Slidercrank (Autodesk Fusion 360 design; units mm, degrees)
Autodesk Fusion 360 part; units mm, degrees
note: some values were not read from the file. Set by a fixed rule: which sketch regions a step uses.
sketch "Sketch2" plane through (0, 0, 0) normal (0, 1, 0) x (1, 0, 0) in component "Bottom"
  circle A0 centre (0, 0) radius 42.5
  dimension "d1" = 85
  constraint coincident A0.centre origin
  measures "d1" diameter of A0
extrude "Extrude1" add sketch "Sketch2" along normal blind 7 makes body 1 in component "Bottom"
sketch "Sketch3" plane through (0, 7, 0) normal (0, 1, 0) x (-1, 0, 0) in component "Bottom"
  circle A0 centre (0, 0) radius 42.5
  circle A1 centre (0, 0) radius 32.5
  circle A2 centre (0, 0) radius 37.5
  dimension "d4" = 65
  dimension "d5" = 75
  constraint coincident A0.centre A1.centre
  constraint concentric A1 A2
  measures "d4" diameter of A1
  measures "d5" diameter of A2
sketch "Sketch1" plane through (0, 7, 0) normal (0, 1, 0) x (-1, 0, 0) in component "Crank1"
  circle A0 centre (35, 0) radius 5
  circle A1 centre (0, 0) radius 42.5
  dimension "d53" = 10
  measures "d53" diameter of A0
extrude "Extrude1'" add sketch "Sketch1" along normal blind 20 separate body contours A0 makes body 2 in component "Crank1"
sketch "Sketch2 (2)" plane through (0, 27, 0) normal (0, 1, 0) x (-1, 0, 0) in component "Crank1"
  circle A0 centre (35, 0) radius 5
  circle A1 centre (35, 0) radius 5
  dimension "d10" = 10
  constraint concentric A0 A1
  measures "d10" diameter of A1
extrude "Extrude2" add sketch "Sketch2 (2)" against normal blind 7.5 bodies 2 in component "Crank1"
extrude "Extrude3" add 1 faces at (-33.6229, 27, 0.9389) along direction (0, 1, 0) blind 5 on bodies 2 bodies 2 in component "Crank1"
ref_plane "WorkPlane1" through (0, 10, 0) normal (0, 1, 0) x (1, 0, 0)
sketch "Sketch3 (2)" plane through (0, 10, 0) normal (0, 1, 0) x (-1, 0, 0) in component "Crank1"
  circle A0 centre (35, 0) radius 5
  line L0 (32.9188, -4.5463) -> (32.9188, 4.5463)
  line L1 (32.9188, 4.5463) -> (-52.0812, 4.5463)
  line L2 (-52.0812, 4.5463) -> (-52.0812, -4.5463)
  line L3 (-52.0812, -4.5463) -> (32.9188, -4.5463)
  circle A1 centre (0, 0) radius 42.5
  point P0 (32.9188, -4.5463)
  point P1 (32.9188, 4.5463)
  dimension "d15" = 85
  constraint coincident A0 P0
  constraint coincident A0 P1
  constraint perpendicular L0 L1
  constraint parallel L0 L2
  constraint parallel L1 L3
  constraint coincident P1 L0.end
  constraint vertical L0
  constraint coincident P0 L0.start
  measures "d15" distance of P0 L2.end
extrude "Extrude4" add sketch "Sketch3 (2)" along normal blind 5 contours A0 L1 L3 A1 | L1 L2 L3 A1 picked at (-18.3153, 0) bodies 2 in component "Crank1"
sketch "Sketch4" plane through (0, 15, 0) normal (0, 1, 0) x (-1, 0, 0) in component "Crank1"
  line L0 (32.9188, 4.5463) -> (-52.0812, 4.5463)
  line L1 (-52.0812, 4.5463) -> (-52.0812, -4.5463)
  line L2 (-52.0812, -4.5463) -> (32.9188, -4.5463)
  circle A0 centre (-52.0812, 0) radius 5
  arc A1 (32.9188, 4.5463) -> (32.9188, -4.5463) centre (35, 0) ccw
  dimension "d18" = 10
  constraint midpoint L1 A0.centre
  measures "d18" diameter of A0
extrude "Extrude5" add sketch "Sketch4" against normal blind 1.5 contours L0 L1 L2 A0 | L0 L1 L2 A0 bodies 2 in component "Crank1"
sketch "Sketch5" plane through (0, 10, 0) normal (0, -1, 0) x (1, 0, 0) in component "Crank1"
  line L0 (-32.9188, -4.5463) -> (52.0812, -4.5463)
  line L1 (52.0812, -4.5463) -> (52.0812, 4.5463)
  line L2 (52.0812, 4.5463) -> (-32.9188, 4.5463)
  circle A0 centre (52.0812, 0) radius 5
  arc A1 (-32.9188, -4.5463) -> (-32.9188, 4.5463) centre (-35, 0) ccw
  dimension "d21" = 10
  constraint midpoint L1 A0.centre
  measures "d21" diameter of A0
extrude "Extrude6" add sketch "Sketch5" against normal blind 1.5 contours L0 L1 L2 A0 | L0 L1 L2 A0 bodies 2 in component "Crank1"
sketch "Sketch6" plane through (0, 11.5, 0) normal (0, 1, 0) x (-1, 0, 0) in component "Crank1"
  line L0 (-52.0812, -4.5463) -> (-52.0812, 4.5463)
  arc A0 (-50, 4.5463) -> (-50, -4.5463) centre (-52.0812, 0) ccw
  circle A1 centre (-52.0812, 0) radius 5
  line L1 (-50, -4.5463) -> (-52.0812, -4.5463)
  line L2 (-52.0812, 4.5463) -> (-50, 4.5463)
  dimension "d24" = 10
  constraint concentric A0 A1
  measures "d24" diameter of A1
extrude "Extrude7" cut sketch "Sketch6" along normal blind 2 bodies 2 in component "Crank1"
sketch "Sketch7" plane through (0, 15, 0) normal (0, 1, 0) x (-1, 0, 0) in component "Crank1"
  line L0 (-50, -4.5463) -> (32.9188, -4.5463)
  line L1 (32.9188, 4.5463) -> (-50, 4.5463)
  arc A0 (-50, 4.5463) -> (-50, -4.5463) centre (-52.0812, 0) ccw
  circle A1 centre (-52.0812, 0) radius 2.5
  arc A2 (32.9188, 4.5463) -> (32.9188, -4.5463) centre (35, 0) ccw
  dimension "d27" = 5
  constraint concentric A0 A1
  measures "d27" diameter of A1
extrude "Extrude8" cut sketch "Sketch7" against normal through all contours A1 bodies 2 in component "Crank1"
sketch "Sketch1 (2)" plane through (0, 11.5, 0) normal (0, 1, 0) x (-1, 0, 0) in component "Crank2"
  circle A0 centre (-52.0812, 0) radius 2.5
  arc A1 (-50, 4.5463) -> (-50, -4.5463) centre (-52.0812, 0) ccw
  arc A2 (-50, -4.5463) -> (-50, 4.5463) centre (-52.0812, 0) ccw
  circle A3 centre (-52.0812, 0) radius 5
  circle A4 centre (-52.0812, 0) radius 2.5
  point P0 (-50.6139, 0)
  point P1 (-50.9156, 0)
  dimension "d29" = 10
  dimension "d30" = 5
  constraint concentric A0 A3
  constraint concentric A3 A4
  measures "d29" diameter of A3
  measures "d30" diameter of A4
extrude "Extrude1''" add sketch "Sketch1 (2)" along normal blind 2 separate body makes body 3 in component "Crank2"
sketch "Sketch2 (3)" plane through (0, 15, 0) normal (0, 1, 0) x (-1, 0, 0) in component "Crank2"
  circle A0 centre (-52.0812, 0) radius 2.5
  line L0 (-50, -4.5463) -> (32.9188, -4.5463)
  line L1 (32.9188, 4.5463) -> (-50, 4.5463)
  arc A1 (-50, 4.5463) -> (-50, -4.5463) centre (-52.0812, 0) ccw
  line L2 (-54.849, -4.164) -> (-54.849, 4.164)
  line L3 (-54.849, 4.164) -> (-154.849, 4.164)
  line L4 (-154.849, 4.164) -> (-154.849, -4.164)
  line L5 (-154.849, -4.164) -> (-54.849, -4.164)
  arc A2 (32.9188, 4.5463) -> (32.9188, -4.5463) centre (35, 0) ccw
  point P0 (-54.849, -4.164)
  point P1 (-54.849, 4.164)
  point P2 (-50.6139, 0)
  point P3 (-50.9156, 0)
  dimension "d33" = 100
  dimension "d34" = 8.328
  constraint coincident A1 P0
  constraint coincident A1 P1
  constraint perpendicular L2 L3
  constraint parallel L2 L4
  constraint parallel L3 L5
  constraint coincident P1 L2.end
  constraint vertical L2
  constraint coincident P0 L2.start
  measures "d33" distance of P0 L4.end
  measures "d34" distance of P0 P1
extrude "Extrude2'" add sketch "Sketch2 (3)" against normal blind 5 contours A1 L3 L4 L5 bodies 3 in component "Crank2"
sketch "Sketch1 (3)" plane through (0, 15, 0) normal (0, 1, 0) x (-1, 0, 0) in component "Linkage stick"
  circle A0 centre (-52.0812, 0) radius 2.5
  line L0 (-50, -4.5463) -> (32.9188, -4.5463)
  line L1 (32.9188, 4.5463) -> (-50, 4.5463)
  arc A1 (-50, 4.5463) -> (-50, -4.5463) centre (-52.0812, 0) ccw
  circle A2 centre (-52.0812, 0) radius 2.5
  arc A3 (32.9188, 4.5463) -> (32.9188, -4.5463) centre (35, 0) ccw
  point P0 (-50.6139, 0)
  point P1 (-50.9156, 0)
  dimension "d37" = 5
  constraint concentric A0 A2
  measures "d37" diameter of A2
extrude "Extrude1'''" add sketch "Sketch1 (3)" along normal blind 2 separate body contours A0 A2 makes body 4 in component "Linkage stick"
extrude "Extrude2''" add 1 faces at (52.7865, 15, -0.2456) along direction (0, -1, 0) blind 7 on bodies 4 bodies 4 in component "Linkage stick"
sketch "Sketch1 (4)" plane through (0, 0, 0) normal (0, 1, 0) x (1, 0, 0) in component "Ground"
  line L0 (135, 10) -> (145, 10)
  line L1 (145, 10) -> (145, -10)
  line L2 (145, -10) -> (135, -10)
  line L3 (135, -10) -> (135, 10)
  dimension "d42" = 135
  dimension "d43" = 10
  dimension "d44" = 20
  dimension "d45" = 10
  constraint horizontal L0
  constraint vertical L1
  constraint horizontal L2
  constraint vertical L3
  measures "d42" distance of origin L3
  measures "d43" distance of L0.start L0.end
  measures "d44" distance of L0.start L2.end
  measures "d45" distance of origin L0
extrude "Extrude1''''" add sketch "Sketch1 (4)" along normal blind 2.5 separate body makes body 5 in component "Ground"
sketch "Sketch2 (4)" plane through (145, 0, 0) normal (1, 0, 0) x (0, 0, -1) in component "Ground"
  line L0 (-10, 0) -> (10, 0)
  line L1 (10, 0) -> (10, 2.5)
  line L2 (10, 2.5) -> (-10, 2.5)
  line L3 (-10, 2.5) -> (-10, 0)
  line L4 (-5, 2.5) -> (5, 2.5)
  line L5 (5, 2.5) -> (5, 14.5)
  line L6 (-5, 14.5) -> (-5, 2.5)
  arc A0 (5, 14.5) -> (-5, 14.5) centre (0, 14.5) ccw
  line L7 (4.164, 15) -> (-4.164, 15)
  line L8 (-4.164, 15) -> (-4.164, 10)
  line L9 (-4.164, 10) -> (4.164, 10)
  line L10 (4.164, 10) -> (4.164, 15)
  line L11 (-4.164, 15) -> (4.164, 15)
  line L12 (4.164, 15) -> (4.164, 10)
  line L13 (4.164, 10) -> (-4.164, 10)
  line L14 (-4.164, 10) -> (-4.164, 15)
  dimension "d48" = 5
  dimension "d49" = 5
  constraint horizontal L4
  constraint vertical L5
  constraint vertical L6
  constraint coincident L2 L4.start
  constraint horizontal L11
  constraint vertical L12
  constraint horizontal L13
  constraint vertical L14
  constraint coincident L9.end L10.start
  constraint coincident L7.end L8.start
  measures "d48" distance of L3 L6
  measures "d49" distance of L1 L5
extrude "Extrude2'''" add sketch "Sketch2 (4)" against normal blind 10 contours L2 L4 L5 L6 A0 bodies 5 in component "Ground"
sketch "Sketch1 (5)" plane through (0, 32, 0) normal (0, 1, 0) x (-1, 0, 0)
  circle A0 centre (35, 0) radius 5
  circle A1 centre (35, 0) radius 7.5
  dimension "d54" = 15
  constraint concentric A0 A1
  measures "d54" diameter of A1
extrude "Extrude9" add sketch "Sketch1 (5)" along normal blind 70 contours A0 | A1 bodies 2 in component "Crank1"
fillet "Fillet1" radius 4 1 edges at (-28.0075, 102, -2.7121) on bodies 2 in component "Crank1"
component "Bottom" placed x (1, 0, 0) y (0, 1, 0) z (0, 0, 1) at (0, 0, 0)
component "Crank1" placed x (1, 0, 0) y (0, 1, 0) z (0, 0, 1) at (0, 0, 0)
component "Crank2" placed x (1, 0, 0) y (0, 1, 0) z (0, 0, 1) at (0, 0, 0)
component "Linkage stick" placed x (1, 0, 0) y (0, 1, 0) z (0, 0, 1) at (0, 0, 0)
component "Ground" placed x (1, 0, 0) y (0, 1, 0) z (0, 0, 1) at (0, 0, 0)
